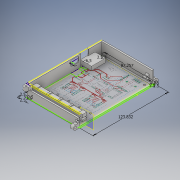
# Autodesk Inventor part: 128chan_box_2_FixedMeasurements
Saved by Autodesk Inventor 2019 (Build 230136000, 136)
## iProperties
Created: 2019-06-17
Part Number: 128chan_box_2_FixedMeasurements
Material: Generic
Document SubType Name: Modeling
Designer: robeyj20
Density: 1 g/cm^3
Appearance: Default
Author: robeyj20
Autodesk Inventor part; units mm, degrees
ref_plane "YZ Plane" through (0, 0, 0) normal (1, 0, 0) x (0, 1, 0)
ref_plane "XZ Plane" through (0, 0, 0) normal (0, 1, 0) x (-1, 0, 0)
ref_plane "XY Plane" through (0, 0, 0) normal (0, 0, 1) x (1, 0, 0)
sketch "Sketch3" plane through (0, 0, 0) normal (0, 1, 0) x (-1, 0, 0)
  line L0 (67.399, 24.8849) -> (69.899, 24.8849)
  line L1 (69.899, 24.8849) -> (69.899, 27.3849)
  line L2 (-9.858, -88.9471) -> (-9.858, -91.4471)
  line L3 (-9.858, -91.4471) -> (-12.358, -91.4471)
  line L4 (-12.358, -91.4471) -> (69.899, -91.4471)
  line L5 (69.899, -91.4471) -> (69.899, 27.3849)
  line L6 (69.899, 27.3849) -> (-12.358, 27.3849)
  line L7 (-12.358, 27.3849) -> (-12.358, -91.4471)
  line L8 (69.899, 27.3849) -> (72.399, 27.3849)
  line L9 (72.399, 27.3849) -> (72.399, 29.8849)
  line L10 (72.399, 29.8849) -> (69.899, 29.8849)
  line L11 (69.899, 29.8849) -> (69.899, 27.3849)
  line L12 (-12.358, -91.4471) -> (-14.858, -91.4471)
  line L13 (-14.858, -91.4471) -> (-14.858, -93.9471)
  line L14 (-14.858, -93.9471) -> (-12.358, -93.9471)
  line L15 (-12.358, -93.9471) -> (-12.358, -91.4471)
  line L16 (72.399, 29.8849) -> (-14.858, 29.8849)
  line L17 (-14.858, 29.8849) -> (-14.858, -93.9471)
  line L18 (-14.858, -93.9471) -> (72.399, -93.9471)
  line L19 (72.399, -93.9471) -> (72.399, 29.8849)
  line L20 (-12.358, 27.3849) -> (-9.858, 27.3849)
  line L21 (-9.858, 27.3849) -> (-9.858, 24.8849)
  line L22 (-9.858, 24.8849) -> (-12.358, 24.8849)
  line L23 (-12.358, 24.8849) -> (-12.358, 27.3849)
  line L24 (-9.858, 24.8849) -> (67.3988, 24.8849) construction
  line L25 (67.3988, 24.8849) -> (67.3988, -88.9472) construction
  line L26 (67.3988, -88.9472) -> (-9.858, -88.9472) construction
  line L27 (-9.858, -88.9472) -> (-9.858, 24.8849) construction
  point P0 (0, 0)
  dimension "d6" = 2.5
  dimension "d7" = 2.5
  dimension "d8" = 2.5
  dimension "d9" = 2.5
  dimension "d10" = 2.5
  dimension "d11" = 2.5
  dimension "d12" = 2.5
  dimension "d13" = 2.5
  dimension "d140" = 123.832
  dimension "d149" = 2.5
  dimension "d150" = 2.5
  dimension "d154" = 87.257
  constraints: 48 end point, 10 parallel, 7 perpendicular, 6 horizontal, 1 vertical, 2 other
  measures "d6" distance of L0.start L0.end
  measures "d7" distance of L0.end L1.end
  measures "d8" distance of L2.start L2.end
  measures "d9" distance of L2.end L3.end
  measures "d10" distance of L10.end L9.end
  measures "d11" distance of L9.end L8.end
  measures "d12" distance of L14.end L13.end
  measures "d13" distance of L13.end L12.end
  measures "d140" distance between parallel lines of L18 L16
  measures "d149" distance of L21.end L22.end
  measures "d150" distance of L20.end L21.end
  measures "d154" distance of L9.end L16.end
extrude "Extrusion1" add sketch "Sketch3" against normal blind 2.5
sketch "Sketch6" plane through (0, 0, 0) normal (0, 1, 0) x (1, 0, 0)
  line L0 (14.858, -29.8849) -> (-72.399, -29.8849) projected
  line L1 (14.858, 93.9471) -> (14.858, -29.8849) projected
  line L2 (-72.399, -29.8849) -> (14.858, -29.8849)
  line L3 (14.858, -29.8849) -> (14.858, -27.3849)
  line L4 (14.858, -27.3849) -> (-72.399, -27.3849)
  line L5 (-72.399, -27.3849) -> (-72.399, -29.8849)
  point P0 (0, 0)
  dimension "d17" = 2.5
  constraints: 8 end point, 2 parallel, 1 horizontal, 1 perpendicular, 1 point on line
  measures "d17" distance of L3.end L2.end
extrude "Extrusion2" add sketch "Sketch6" along normal blind 19.5
sketch "Sketch7" plane through (0, 0, 0) normal (0, 1, 0) x (1, 0, 0)
  point P0 (0, 0)
sketch "Sketch8" plane through (0, 0, 0) normal (0, 1, 0) x (1, 0, 0)
  line L0 (-72.399, 93.9471) -> (14.858, 93.9471) projected
  line L1 (14.858, -27.3849) -> (-72.399, -27.3849) projected
  line L2 (14.858, 93.9471) -> (12.358, 93.9471)
  line L3 (12.358, 93.9471) -> (12.358, -27.3849)
  line L4 (12.358, -27.3849) -> (14.858, -27.3849)
  line L5 (14.858, -27.3849) -> (14.858, 93.9471)
  line L6 (-72.399, -29.8849) -> (-72.399, 93.9471) projected
  line L7 (12.358, 93.9471) -> (-72.399, 93.9471)
  line L8 (-72.399, 93.9471) -> (-72.399, 91.4471)
  line L9 (-72.399, 91.4471) -> (12.358, 91.4471)
  line L10 (12.358, 91.4471) -> (12.358, 93.9471)
  point P0 (0, 0)
  dimension "d20" = 2.5
  dimension "d21" = 2.5
  constraints: 16 end point, 4 parallel, 2 horizontal, 2 perpendicular, 2 point on line
  measures "d20" distance of L4.end L3.end
  measures "d21" distance of L8.end L7.end
extrude "Extrusion3" add sketch "Sketch8" along normal blind 19.5 contours L0 L3 L9 L6 | L0 L5 L1 L3
sketch "Sketch9" plane through (0, 0, 0) normal (0, 1, 0) x (1, 0, 0)
  circle A0 centre (7.2566, -20.3487) radius 1.4722
  point P0 (0, 0)
  constraints: 1 centre point
extrude "Extrusion4" cut sketch "Sketch9" against normal through all
sketch "Sketch10" plane through (0, 0, 0) normal (0, 1, 0) x (1, 0, 0)
  circle A0 centre (-64.6728, -20.3503) radius 1.5
  point P0 (0, 0)
  dimension "d26" = 3
  constraints: 1 centre point
  measures "d26" diameter of A0
extrude "Extrusion5" cut sketch "Sketch10" against normal blind 15.5
sketch "Sketch11" plane through (0, 0, 0) normal (0, 1, 0) x (1, 0, 0)
  circle A0 centre (-64.6729, 76.3591) radius 1.5
  point P0 (0, 0)
  dimension "d29" = 3
  constraints: 1 centre point
  measures "d29" diameter of A0
extrude "Extrusion6" cut sketch "Sketch11" against normal blind 15.5
sketch "Sketch12" plane through (0, 0, 0) normal (0, 1, 0) x (1, 0, 0)
  circle A0 centre (7.2293, 76.3561) radius 1.5
  point P0 (0, 0)
  dimension "d32" = 3
  constraints: 1 centre point
  measures "d32" diameter of A0
extrude "Extrusion7" cut sketch "Sketch12" against normal blind 15.5
sketch "Sketch17" plane through (0, 0, 0) normal (0, 1, 0) x (1, 0, 0)
  line L0 (5.4643, -3.3659) -> (5.4643, 6.7846)
  line L1 (5.4643, 6.7846) -> (9.8324, 6.7846)
  line L2 (5.4643, -3.3659) -> (9.8324, -3.3659)
  line L3 (9.8324, -3.3659) -> (9.8324, 6.7846)
  line L4 (9.8324, 6.7846) -> (12.358, 6.7846)
  line L5 (12.358, 91.4471) -> (12.358, -27.3849) projected
  line L6 (9.8324, -3.3659) -> (12.358, -3.3659)
  line L7 (12.358, -3.3659) -> (12.358, 6.7846)
  line L8 (12.358, 6.7846) -> (18.858, 6.7846)
  line L9 (18.858, 6.7846) -> (18.858, -3.3659)
  line L10 (18.858, -3.3659) -> (12.358, -3.3659)
  line L11 (12.358, -3.3659) -> (12.358, 6.7846)
  line L12 (18.858, -3.3659) -> (27.858, -3.3659)
  line L13 (27.858, -3.3659) -> (27.858, 6.7846)
  line L14 (27.858, 6.7846) -> (18.858, 6.7846)
  line L15 (18.858, 6.7846) -> (18.858, -3.3659)
  point P0 (0, 0)
  dimension "d41" = 6.5
  dimension "d42" = 9
  constraints: 30 end point, 6 perpendicular, 4 parallel, 3 horizontal, 3 point on line, 1 vertical
  measures "d41" distance of L9.end L10.end
  measures "d42" distance of L14.end L13.end
sketch "Sketch18" plane through (12.358, 0, -91.4471) normal (-1, 0, 0) x (0, 0, 1)
  line L0 (97.332, 0) -> (84.332, 0)
  line L1 (84.332, 0) -> (84.332, 10.3)
  line L2 (84.332, 10.3) -> (97.332, 10.3)
  line L3 (97.332, 10.3) -> (97.332, 0)
  line L4 (97.332, 10.3) -> (84.332, 10.3)
  line L5 (84.332, 10.3) -> (84.332, 20.5)
  line L6 (84.332, 20.5) -> (97.332, 20.5)
  line L7 (97.332, 20.5) -> (97.332, 10.3)
  line L8 (121.332, -2.5) -> (121.332, 19.5) projected
  point P0 (91.4471, 0)
  dimension "d43" = 10.3
  dimension "d44" = 10.2
  dimension "d214" = 37
  dimension "d215" = 24
  constraints: 16 end point, 4 parallel, 2 horizontal, 2 perpendicular, 1 point on line
  measures "d43" distance of L0.end L1.end
  measures "d44" distance of L4.end L5.end
  measures "d214" distance between parallel lines of L5 L8
  measures "d215" distance between parallel lines of L8 L7
extrude "Extrusion8" cut sketch "Sketch18" against normal blind 7 contours L2 L5 L6 L7
sketch "Sketch19" plane through (0, 0, 0) normal (0, 1, 0) x (1, 0, 0)
  line L0 (12.358, 91.4471) -> (12.358, -27.3849) projected
  line L1 (12.358, -16.2033) -> (-5.101, -16.2033)
  line L2 (-5.101, -16.2033) -> (-5.101, 6.9014)
  line L3 (-5.101, 6.9014) -> (12.358, 6.9014)
  line L4 (12.358, 6.9014) -> (12.358, -16.2033)
  point P0 (0, 0)
  constraints: 8 end point, 2 parallel, 1 horizontal, 1 perpendicular, 1 point on line
extrude "Extrusion9" add sketch "Sketch19" along normal blind 10.3
sketch "Sketch20" plane through (0, 0, 0) normal (0, 1, 0) x (1, 0, 0)
  line L0 (12.358, 6.9014) -> (12.358, 91.4471) projected
  line L1 (2.9551, 10.786) -> (12.358, 10.786)
  line L2 (12.358, 10.786) -> (12.358, 23.7884)
  line L3 (12.358, 23.7884) -> (2.9551, 23.7884)
  line L4 (2.9551, 23.7884) -> (2.9551, 10.786)
  point P0 (0, 0)
  constraints: 8 end point, 2 parallel, 1 horizontal, 1 perpendicular, 1 point on line
sketch "Sketch22" plane through (12.358, 0, 27.3849) normal (-1, 0, 0) x (0, 0, 1)
  line L0 (-34.2863, 0) -> (-118.832, 0) projected
  line L1 (-37.9099, 0) -> (-50.6984, 0)
  line L2 (-50.6984, 0) -> (-50.6984, 9)
  line L3 (-50.6984, 9) -> (-37.9099, 9)
  line L4 (-37.9099, 9) -> (-37.9099, 0)
  line L5 (-50.6984, 9) -> (-37.9099, 9)
  line L6 (-37.9099, 9) -> (-37.9099, 18)
  line L7 (-37.9099, 18) -> (-50.6984, 18)
  line L8 (-50.6984, 18) -> (-50.6984, 9)
  point P0 (-27.3849, 0)
  dimension "d49" = 9
  dimension "d50" = 9
  constraints: 16 end point, 4 parallel, 2 horizontal, 2 perpendicular, 2 point on line
  measures "d49" distance of L1.end L2.end
  measures "d50" distance of L6.end L5.end
extrude "Extrusion10" cut sketch "Sketch22" against normal blind 7 contours L3 L8 L7 L6
sketch "Sketch27" plane through (-5.101, 0, -6.9014) normal (-1, 0, 0) x (0, 0, 1)
  line L0 (23.1047, 10.3) -> (23.1047, 0) projected
  line L1 (0, 0) -> (0, 10.3) projected
  line L2 (23.1047, 0) -> (0, 0)
  line L3 (0, 0) -> (0, 4)
  line L4 (0, 4) -> (23.1047, 4)
  line L5 (23.1047, 4) -> (23.1047, 0)
  point P0 (6.9014, 0)
  dimension "d53" = 4
  constraints: 8 end point, 2 parallel, 1 horizontal, 1 perpendicular, 1 point on line
  measures "d53" distance of L2.end L3.end
extrude "Extrusion11" cut sketch "Sketch27" against normal blind 17.459
sketch "Sketch28" plane through (0, 0, 0) normal (0, 1, 0) x (1, 0, 0)
  circle A0 centre (-7.2339, 64.144) radius 1.5
  point P0 (0, 0)
  dimension "d56" = 3
  constraints: 1 centre point
  measures "d56" diameter of A0
extrude "Extrusion12" cut sketch "Sketch28" against normal blind 17.459
sketch "Sketch29" plane through (0, 0, 0) normal (0, 1, 0) x (1, 0, 0)
  circle A0 centre (-25.1712, 64.1283) radius 1.5
  point P0 (0, 0)
  dimension "d59" = 3
  constraints: 1 centre point
  measures "d59" diameter of A0
extrude "Extrusion13" cut sketch "Sketch29" against normal blind 17.459
sketch "Sketch31" plane through (0, 0, 0) normal (0, 1, 0) x (1, 0, 0)
  circle A0 centre (-42.8452, 64.1372) radius 1.5
  point P0 (0, 0)
  dimension "d62" = 3
  constraints: 1 centre point
  measures "d62" diameter of A0
extrude "Extrusion14" cut sketch "Sketch31" against normal blind 17.459
sketch "Sketch32" plane through (0, 0, 0) normal (0, 1, 0) x (1, 0, 0)
  circle A0 centre (-60.6502, 64.1297) radius 1.5
  point P0 (0, 0)
  dimension "d65" = 3
  constraints: 1 centre point
  measures "d65" diameter of A0
extrude "Extrusion15" cut sketch "Sketch32" against normal blind 17.459
sketch "Sketch33" plane through (0, 0, 0) normal (0, 1, 0) x (1, 0, 0)
  circle A0 centre (-7.2339, 64.144) radius 1.5 projected
  line L0 (-7.2339, 65.644) -> (9.8529, 65.644)
  line L1 (9.8529, 65.644) -> (12.358, 65.644)
  line L2 (12.358, 6.9014) -> (12.358, 91.4471) projected
  line L3 (12.358, 79.4521) -> (-72.2997, 79.4521)
  line L4 (-72.2997, 79.4521) -> (-72.2997, 86.4521)
  line L5 (-72.2997, 86.4521) -> (12.358, 86.4521)
  line L6 (12.358, 86.4521) -> (12.358, 79.4521)
  point P0 (0, 0)
  dimension "d166" = 7
  dimension "d167" = 84.6577
  constraints: 12 end point, 4 horizontal, 3 point on line, 2 parallel, 1 perpendicular, 1 vertical alignment, 1 other
  measures "d166" distance of L3.end L4.end
  measures "d167" distance of L3.start L3.end
extrude "Extrusion16" add sketch "Sketch33" along normal blind 12.9 contours L3 L4 L5 L2
sketch "Sketch34" plane through (-72.2997, 0, -86.4521) normal (-1, 0, 0) x (0, 0, 1)
  line L0 (7, 0) -> (0, 0) projected
  line L1 (0, 0) -> (0, 12.9) projected
  line L2 (7, 0) -> (0, 0)
  line L3 (0, 0) -> (0, 4)
  line L4 (0, 4) -> (7, 4)
  line L5 (7, 4) -> (7, 0)
  point P0 (86.4521, 0)
  dimension "d70" = 4
  constraints: 8 end point, 2 parallel, 1 horizontal, 1 perpendicular, 1 point on line
  measures "d70" distance of L2.end L3.end
extrude "Extrusion17" cut sketch "Sketch34" against normal blind 84.658
sketch "Sketch40" plane through (14.858, -2.5, -93.9471) normal (0, 0, -1) x (-1, 0, 0)
  line L0 (0, 0) -> (0, 22) projected
  line L1 (2.5, 2.5) -> (87.257, 2.5) projected
  line L2 (87.257, 0) -> (0, 0) projected
  line L3 (0, 0) -> (9, 0)
  line L4 (9, 0) -> (9, 15)
  line L5 (9, 15) -> (0, 15)
  line L6 (0, 15) -> (0, 0)
  line L7 (87.257, 22) -> (2.5, 22) projected
  line L8 (87.257, 22) -> (80.757, 22)
  line L9 (80.757, 22) -> (80.757, 18)
  line L10 (80.757, 18) -> (87.257, 18)
  line L11 (87.257, 18) -> (87.257, 22)
  line L12 (9, 15) -> (80.757, 15)
  line L13 (80.757, 15) -> (80.757, 18)
  line L14 (80.757, 18) -> (9, 18)
  line L15 (9, 18) -> (9, 15)
  dimension "d168" = 4
  dimension "d169" = 15
  dimension "d170" = 6.5
  dimension "d171" = 9
  constraints: 24 end point, 6 parallel, 3 horizontal, 3 perpendicular
  measures "d168" distance of L8.end L9.end
  measures "d169" distance of L3.end L4.end
  measures "d170" distance of L9.end L10.end
  measures "d171" distance of L4.end L5.end
extrude "Extrusion18" cut sketch "Sketch40" against normal blind 5 contours L15 L14 L13 L12
sketch "Sketch42" plane through (-72.399, 0, 27.3849) normal (-1, 0, 0) x (0, 0, 1)
  point P0 (-27.3849, 0)
sketch "Sketch47" plane through (0, 19.5, 0) normal (0, 1, 0) x (1, 0, 0)
  line L0 (-72.399, 93.9471) -> (14.858, 93.9471) projected
  line L1 (14.858, 93.9471) -> (7.358, 93.9471)
  line L2 (7.358, 93.9471) -> (14.858, 93.9471)
  line L3 (14.858, 93.9471) -> (14.858, -29.8849) projected
  line L4 (-72.399, 91.4471) -> (12.358, 91.4471) projected
  line L5 (14.858, 93.9471) -> (12.358, 93.9471)
  line L6 (12.358, 93.9471) -> (12.358, 91.4471)
  line L7 (12.358, 91.4471) -> (14.858, 91.4471)
  line L8 (14.858, 91.4471) -> (14.858, 93.9471)
  line L9 (12.358, 91.4471) -> (16.108, 91.4471) construction
  constraints: 14 end point, 3 horizontal, 2 parallel, 1 perpendicular
sketch "Sketch51" plane through (-72.399, -2.5, -93.9471) normal (-1, 0, 0) x (0, 0, 1)
  point P0 (93.9471, 2.5)
sketch "Sketch55" plane through (0, 19.5, 0) normal (0, 1, 0) x (1, 0, 0)
  line L0 (-72.399, -29.8849) -> (-72.399, 93.9471) projected
  line L1 (-72.399, 93.9471) -> (-69.899, 93.9471)
  line L2 (-69.899, 93.9471) -> (-69.899, -45.8172)
  line L3 (-69.899, -45.8172) -> (-72.399, -45.8172)
  line L4 (-72.399, -45.8172) -> (-72.399, 93.9471)
  point P0 (0, 0)
  point P1 (-72.399, -31.1349)
  dimension "d125" = 2.5
  constraints: 8 end point, 2 parallel, 1 horizontal, 1 perpendicular
  measures "d125" distance of L2.end L3.end
extrude "Extrusion29" cut sketch "Sketch55" against normal through all
sketch "Sketch72" plane through (0, 0, 0) normal (0, 1, 0) x (1, 0, 0)
  line L0 (-69.899, -27.3849) -> (-69.899, -29.8849) projected
  line L1 (-69.899, -27.3849) -> (-64.899, -27.3849)
  line L2 (-64.899, -27.3849) -> (-64.899, -22.3849)
  line L3 (-64.899, -22.3849) -> (-69.899, -22.3849)
  line L4 (-69.899, -22.3849) -> (-69.899, -27.3849)
  line L5 (12.358, -27.3849) -> (-69.899, -27.3849) projected
  line L6 (-64.899, -22.3849) -> (-59.899, -22.3849)
  line L7 (-59.899, -22.3849) -> (-59.899, -27.3849)
  line L8 (-59.899, -27.3849) -> (-64.899, -27.3849)
  line L9 (-64.899, -27.3849) -> (-64.899, -22.3849)
  point P0 (0, 0)
  dimension "d225" = 5
  dimension "d226" = 5
  dimension "d227" = 5
  constraints: 16 end point, 4 parallel, 2 horizontal, 2 perpendicular, 1 point on line
  measures "d225" distance of L3.end L2.end
  measures "d226" distance of L2.end L1.end
  measures "d227" distance of L7.end L8.end
extrude "Extrusion43" add sketch "Sketch72" along normal blind 10 contours L2 L6 L7 L5
sketch "Sketch73" plane through (-64.899, 0, 22.3849) normal (-1, 0, 0) x (0, 0, 1)
  line L0 (5, 0) -> (-6.1817, 0) projected
  line L1 (0, 0) -> (0, 10) projected
  line L2 (5, 0) -> (0, 0)
  line L3 (0, 0) -> (0, 5)
  line L4 (0, 5) -> (5, 5)
  line L5 (5, 5) -> (5, 0)
  point P0 (-22.3849, 0)
  constraints: 8 end point, 2 parallel, 1 horizontal, 1 midpoint, 1 perpendicular
extrude "Extrusion44" cut sketch "Sketch73" against normal blind 10
sketch "Sketch74" plane through (-64.899, 10, 22.3849) normal (-1, 0, 0) x (0, 0, 1)
  circle A0 centre (2.5093, -2.5) radius 1.75
  point P0 (-22.3849, -10)
  dimension "d232" = 3.5
  constraints: 1 centre point
  measures "d232" diameter of A0
extrude "Extrusion45" cut sketch "Sketch74" against normal blind 10
fillet "Fillet15" radius 2 4 edges at (-62.399, 10, 22.3849) (-62.399, 5, 22.3849) (-62.399, 10, 27.3849) (-62.399, 5, 27.3849)
sketch "Sketch75" plane through (0, 12.9, 0) normal (0, 1, 0) x (1, 0, 0)
  line L0 (-69.899, 79.4521) -> (12.358, 79.4521) projected
  line L1 (12.358, 86.4521) -> (-69.899, 86.4521) projected
  line L2 (-69.899, 79.4521) -> (-63.649, 79.4521)
  line L3 (-63.649, 79.4521) -> (-63.649, 86.4521)
  line L4 (-63.649, 86.4521) -> (-69.899, 86.4521)
  line L5 (-69.899, 86.4521) -> (-69.899, 79.4521)
  line L6 (-63.649, 86.4521) -> (-48.399, 86.4521)
  line L7 (-48.399, 86.4521) -> (-48.399, 79.4521)
  line L8 (-48.399, 79.4521) -> (-63.649, 79.4521)
  line L9 (-63.649, 79.4521) -> (-63.649, 86.4521)
  line L10 (-48.399, 79.4521) -> (-46.249, 79.4521)
  line L11 (-46.249, 79.4521) -> (-46.249, 86.4521)
  line L12 (-46.249, 86.4521) -> (-48.399, 86.4521)
  line L13 (-48.399, 86.4521) -> (-48.399, 79.4521)
  line L14 (-46.249, 79.4521) -> (-30.999, 79.4521)
  line L15 (-30.999, 79.4521) -> (-30.999, 86.4521)
  line L16 (-30.999, 86.4521) -> (-46.249, 86.4521)
  line L17 (-46.249, 86.4521) -> (-46.249, 79.4521)
  line L18 (-30.999, 86.4521) -> (-28.809, 86.4521)
  line L19 (-28.809, 86.4521) -> (-28.809, 79.4521)
  line L20 (-28.809, 79.4521) -> (-30.999, 79.4521)
  line L21 (-30.999, 79.4521) -> (-30.999, 86.4521)
  line L22 (-28.809, 86.4521) -> (-13.559, 86.4521)
  line L23 (-13.559, 86.4521) -> (-13.559, 79.4521)
  line L24 (-13.559, 79.4521) -> (-28.809, 79.4521)
  line L25 (-28.809, 79.4521) -> (-28.809, 86.4521)
  line L26 (-13.559, 86.4521) -> (-10.659, 86.4521)
  line L27 (-10.659, 86.4521) -> (-10.659, 79.4521)
  line L28 (-10.659, 79.4521) -> (-13.559, 79.4521)
  line L29 (-13.559, 79.4521) -> (-13.559, 86.4521)
  line L30 (-10.659, 86.4521) -> (4.591, 86.4521)
  line L31 (4.591, 86.4521) -> (4.591, 79.4521)
  line L32 (4.591, 79.4521) -> (-10.659, 79.4521)
  line L33 (-10.659, 79.4521) -> (-10.659, 86.4521)
  line L34 (12.358, 91.4471) -> (12.358, 7.1151) projected
  line L35 (4.591, 79.4521) -> (12.358, 79.4521)
  line L36 (12.358, 79.4521) -> (12.358, 86.4521)
  line L37 (12.358, 86.4521) -> (4.591, 86.4521)
  line L38 (4.591, 86.4521) -> (4.591, 79.4521)
  point P0 (0, 0)
  dimension "d236" = 6.25
  dimension "d237" = 15.25
  dimension "d238" = 2.15
  dimension "d239" = 15.25
  dimension "d240" = 2.19
  dimension "d241" = 15.25
  dimension "d242" = 2.9
  dimension "d243" = 15.25
  constraints: 72 end point, 18 parallel, 10 point on line, 9 horizontal, 9 perpendicular
  measures "d236" distance of L4.end L3.end
  measures "d237" distance of L7.end L8.end
  measures "d238" distance of L12.end L11.end
  measures "d239" distance of L16.end L15.end
  measures "d240" distance of L19.end L20.end
  measures "d241" distance of L23.end L24.end
  measures "d242" distance of L27.end L28.end
  measures "d243" distance of L31.end L32.end
extrude "Extrusion46" add sketch "Sketch75" along normal blind 1.25 contours L5 L1 L3 L0 | L7 L1 L11 L0 | L15 L1 L19 L0 | L23 L1 L27 L0 | L31 L1 L34 L0
fillet "Fillet9" radius 1.5 17 edges at (14.858, 8.5, 29.8849) (-27.5205, -2.5, 29.8849) (14.858, -2.5, -32.0311) (14.858, 8.5, -93.9471) (13.608, 9, -10.525) (13.608, 18, -10.525) (13.608, 18, -23.3134) (13.608, 9, -23.3134) (14.858, 14.9, -7.1151) (14.858, 14.9, 5.8849) (14.858, 10.3, -0.6151) (13.608, 10.3, 5.8849) (14.858, 13.5, -23.3134) (14.858, 18, -16.9192) (14.858, 13.5, -10.525) (-28.7705, 0, 27.3849) (14.858, 9, -16.9192)
sketch "Sketch60" plane through (-69.899, 0, 27.3849) normal (-1, 0, 0) x (0, 0, 1)
  line L0 (1, -2.5) -> (-121.332, -2.5) projected
  line L1 (-121.332, -2.5) -> (-125.082, -2.5)
  line L2 (-125.082, -2.5) -> (-125.082, 1.25)
  line L3 (-125.082, 1.25) -> (-121.332, 1.25)
  line L4 (-121.332, 1.25) -> (-121.332, -2.5)
  circle A0 centre (-125.082, 1.25) radius 3.75
  line L5 (-121.332, -2.5) -> (-125.082, -2.5)
  line L6 (-125.082, 5) -> (-121.332, 5)
  line L7 (-121.332, 5) -> (-121.332, -2.5)
  line L8 (-121.332, -2.5) -> (-125.082, -2.5)
  line L9 (-125.082, -2.5) -> (-125.082, 5)
  line L10 (-125.082, 5) -> (-121.332, 5)
  line L11 (-121.332, 5) -> (-121.332, -2.5)
  circle A1 centre (-125.082, 1.25) radius 1.5
  point P0 (-27.3849, 0)
  point P1 (3.75, -2.5)
  dimension "d184" = 7.5
  dimension "d182" = 3.75
  dimension "d183" = 3.75
  dimension "d188" = 3
  constraints: 22 end point, 5 parallel, 3 horizontal, 2 coincident, 2 perpendicular, 1 centre point, 1 vertical alignment, 2 other
  measures "d182" distance of L2.end L3.end
  measures "d183" distance of L1.end L2.end
  measures "d188" diameter of A1
extrude "Extrusion32" add sketch "Sketch60" against normal blind 5
sketch "Sketch61" plane through (-69.899, 0, 27.3849) normal (-1, 0, 0) x (0, 0, 1)
  line L0 (-119.9922, 10.5) -> (-119.9922, 11) projected
  line L1 (-121.3234, -2.4914) -> (-125.0734, -2.4914)
  line L2 (-125.0734, -2.4914) -> (-125.0734, 1.2586)
  line L3 (-125.0734, 1.2586) -> (-121.3234, 1.2586)
  line L4 (-121.3234, 1.2586) -> (-121.3234, -2.4914)
  circle A0 centre (-125.0734, 1.2586) radius 1.5
  point P0 (-27.3849, 0)
  point P1 (-121.3234, 11)
  point P2 (-121.3234, 19.5)
  dimension "d189" = 3.75
  dimension "d190" = 3.75
  dimension "d191" = 3
  constraints: 8 end point, 2 parallel, 1 centre point, 1 coincident, 1 horizontal, 1 perpendicular, 1 other
  measures "d189" distance of L2.end L3.end
  measures "d190" distance of L1.end L2.end
  measures "d191" diameter of A0
extrude "Extrusion33" cut sketch "Sketch61" against normal blind 5 contours A0 L3 L2 | L2 L3 A0
sketch "Sketch62" plane through (-69.899, 0, -91.4471) normal (-1, 0, 0) x (0, 0, 1)
  arc A0 (119.832, -2.5) -> (121.332, -1) centre (119.832, -1) ccw projected
  line L0 (119.832, -2.5) -> (121.332, -2.5)
  line L1 (121.332, -2.5) -> (125.082, -2.5)
  line L2 (125.082, -2.5) -> (125.082, 5)
  line L3 (125.082, 5) -> (121.332, 5)
  line L4 (121.332, 5) -> (121.332, -2.5)
  circle A1 centre (125.082, 1.25) radius 3.75
  point P0 (91.4471, 0)
  dimension "d194" = 3.75
  dimension "d195" = 7.5
  constraints: 10 end point, 2 horizontal, 2 parallel, 1 midpoint, 1 perpendicular, 1 tangent, 1 vertical alignment, 2 other
  measures "d194" distance of L3.end L2.end
  measures "d195" distance of L2.end L1.end
extrude "Extrusion34" add sketch "Sketch62" against normal blind 5 contours L4 A1 L1 | L4 L3 A1 | A1 L2 | L2 A1
sketch "Sketch63" plane through (-69.899, 0, -91.4471) normal (-1, 0, 0) x (0, 0, 1)
  line L0 (121.332, -2.5) -> (125.082, -2.5) projected
  line L1 (-1, -1) -> (119.832, -1) projected
  line L2 (121.332, -2.5) -> (119.832, -2.5)
  line L3 (119.832, -2.5) -> (119.832, -1)
  line L4 (119.832, -1) -> (121.332, -1)
  line L5 (121.332, -1) -> (121.332, -2.5)
  point P0 (91.4471, 0)
  constraints: 8 end point, 2 parallel, 1 horizontal, 1 perpendicular
extrude "Extrusion35" add sketch "Sketch63" against normal blind 5
sketch "Sketch64" plane through (-69.899, 0, -91.4471) normal (-1, 0, 0) x (0, 0, 1)
  arc A0 (125.082, -2.5) -> (125.082, 5) centre (125.082, 1.25) ccw projected
  circle A1 centre (125.082, 1.25) radius 1.5
  point P0 (91.4471, 0)
  dimension "d200" = 3
  constraints: 1 centre point, 1 coincident
  measures "d200" diameter of A1
extrude "Extrusion36" cut sketch "Sketch64" against normal blind 5
sketch "Sketch65" plane through (0, 19.5, 0) normal (0, 1, 0) x (1, 0, 0)
  line L0 (14.858, 93.9471) -> (7.358, 93.9471)
  line L1 (7.358, 93.9471) -> (7.358, 97.6971)
  line L2 (7.358, 97.6971) -> (14.858, 97.6971)
  line L3 (14.858, 97.6971) -> (14.858, 93.9471)
  circle A0 centre (11.108, 97.6971) radius 3.75
  point P0 (0, 0)
  dimension "d203" = 7.5
  dimension "d204" = 3.75
  dimension "d205" = 7.5
  constraints: 8 end point, 2 parallel, 1 centre point, 1 horizontal, 1 midpoint, 1 perpendicular
  measures "d203" distance of L1.end L2.end
  measures "d204" distance of L0.end L1.end
  measures "d205" diameter of A0
extrude "Extrusion37" add sketch "Sketch65" against normal blind 5
sketch "Sketch66" plane through (0, 19.5, 0) normal (0, 1, 0) x (1, 0, 0)
  arc A0 (14.858, 97.6971) -> (7.358, 97.6971) centre (11.108, 97.6971) ccw projected
  circle A1 centre (11.108, 97.6971) radius 1.5
  point P0 (0, 0)
  dimension "d208" = 3
  constraints: 1 centre point, 1 coincident
  measures "d208" diameter of A1
extrude "Extrusion38" cut sketch "Sketch66" against normal blind 5
sketch "Sketch67" plane through (0, 19.5, 0) normal (0, 1, 0) x (1, 0, 0)
  line L0 (-69.899, 91.4471) -> (12.358, 91.4471) projected
  line L1 (14.858, 93.9471) -> (13.358, 93.9471) projected
  line L2 (12.358, 91.4471) -> (14.858, 91.4471)
  line L3 (14.858, 91.4471) -> (14.858, 93.9471)
  line L4 (14.858, 93.9471) -> (12.358, 93.9471)
  line L5 (12.358, 93.9471) -> (12.358, 91.4471)
  point P0 (0, 0)
  constraints: 8 end point, 2 parallel, 1 horizontal, 1 perpendicular
extrude "Extrusion39" add sketch "Sketch67" against normal blind 5
fillet "Fillet14" radius 1.5 2 edges at (-25.7704, -2.5, -93.9471) (14.4187, -2.0607, -93.5078)
sketch "Sketch68" plane through (-64.899, 5, -93.9471) normal (0, 0, -1) x (-1, 0, 0)
  line L0 (-70.757, 7.5) -> (1, 7.5) projected
  line L1 (5, 14.5) -> (5, 0) projected
  line L2 (-70.757, 7.5) -> (5, 7.5)
  line L3 (5, 7.5) -> (5, 14.5)
  line L4 (5, 14.5) -> (-70.757, 14.5)
  line L5 (-70.757, 14.5) -> (-70.757, 7.5)
  line L6 (-72.257, 14.5) -> (-72.257, 9.5) projected
  line L7 (-70.757, 7.5) -> (-72.257, 7.5)
  line L8 (-72.257, 7.5) -> (-72.257, 14.5)
  line L9 (-72.257, 14.5) -> (-70.757, 14.5)
  line L10 (-70.757, 14.5) -> (-70.757, 7.5)
  point P0 (-64.899, -5)
  constraints: 16 end point, 4 parallel, 2 horizontal, 2 perpendicular
extrude "Extrusion40" cut sketch "Sketch68" against normal blind 2.5
ref_plane "Work Plane2" through (-69.899, 5, -79.4521) normal (0, 0, 1) x (1, 0, 0)
sketch "Sketch69" plane through (-69.899, 5, -79.4521) normal (0, 0, 1) x (1, 0, 0)
  line L0 (82.257, 0) -> (0, 0) projected
  line L1 (0, 0) -> (6.172, 0)
  line L2 (0, 1.2219) -> (3, 1.2219)
  line L3 (3, 1.2219) -> (3, 4.2219)
  line L4 (3, 4.2219) -> (0, 4.2219)
  line L5 (0, 4.2219) -> (0, 1.2219)
  circle A0 centre (3, 2.7219) radius 1.5
  point P0 (69.899, -5)
  dimension "d221" = 3
  dimension "d222" = 3
  constraints: 10 end point, 2 horizontal, 2 parallel, 1 midpoint, 1 perpendicular, 1 vertical alignment, 2 other
  measures "d221" distance of L4.end L3.end
  measures "d222" distance of L3.end L2.end
extrude "Extrusion42" cut sketch "Sketch69" against normal through all
body "Solid1"
